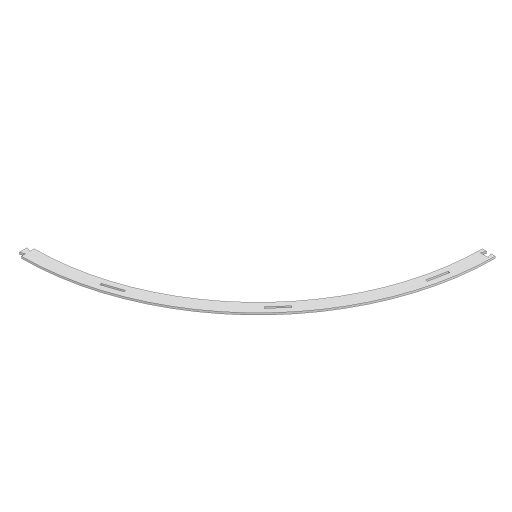
# Autodesk Inventor part: R70_CM_CIRCULO
Saved by Autodesk Inventor 2024.2 (Build 282272000, 272)
## iProperties
Created: 2024-10-01
Part Number: R70_CM_CIRCULO
Material: Generic
Document SubType Name: Modeling
Designer: jrcer
Density: 1 g/cm^3
Appearance: Default
Author: jrcer
Autodesk Inventor part; units mm, degrees
ref_plane "YZ Plane" through (0, 0, 0) normal (1, 0, 0) x (0, 1, 0)
ref_plane "XZ Plane" through (0, 0, 0) normal (0, 1, 0) x (-1, 0, 0)
ref_plane "XY Plane" through (0, 0, 0) normal (0, 0, 1) x (1, 0, 0)
sketch "Sketch1" plane through (0, 0, 0) normal (0, 1, 0) x (-1, 0, 0)
  circle A0 centre (0, 0) radius 350
  circle A1 centre (0, 0) radius 370
  line L0 (370, 0) -> (350, 0)
  line L1 (-370, 0) -> (-350, 0)
  line L2 (0, 0) -> (-350, 0) construction
  line L3 (0, 350) -> (0, 0) construction
  line L4 (0, 370) -> (0, 350)
  line L5 (-350, 0) -> (-370, 0)
  line L6 (-354, 7) -> (-366, 7)
  line L7 (-366, 7) -> (-363.4522, 0)
  line L8 (-354, 7) -> (-356.5478, 0)
  line L9 (-360, 0) -> (-360, 7) construction
  line L10 (-356.9749, 57.6407) -> (-350.9683, 87.0332)
  line L11 (-350.9683, 87.0332) -> (-347.8331, 86.3925)
  line L12 (-347.8331, 86.3925) -> (-353.8397, 57)
  line L13 (-353.8397, 57) -> (-356.9749, 57.6407)
  line L14 (-356.9749, 57.6407) -> (-347.8331, 86.3925) construction
  line L15 (-350.9683, 87.0332) -> (-353.8397, 57) construction
  circle A2 centre (0, 0) radius 360 construction
  line L16 (-7, -354) -> (0, -356.5478)
  line L17 (-7, -366) -> (0, -363.4522)
  line L18 (-7, -354) -> (-7, -366)
  line L19 (354, -7) -> (356.5478, 0)
  line L20 (366, -7) -> (363.4522, 0)
  line L21 (354, -7) -> (366, -7)
  line L22 (7, 354) -> (0, 356.5478)
  line L23 (7, 366) -> (0, 363.4522)
  line L24 (7, 354) -> (7, 366)
  line L25 (-337.9697, -128.5692) -> (-347.4641, -100.1112)
  line L26 (-334.9342, -127.5564) -> (-337.9697, -128.5692)
  line L27 (-344.4286, -99.0984) -> (-334.9342, -127.5564)
  line L28 (-347.4641, -100.1112) -> (-344.4286, -99.0984)
  line L29 (-228.4058, -280.329) -> (-250.8572, -260.4309)
  line L30 (-226.2833, -277.9342) -> (-228.4058, -280.329)
  line L31 (-248.7347, -258.0361) -> (-226.2833, -277.9342)
  line L32 (-250.8572, -260.4309) -> (-248.7347, -258.0361)
  line L33 (-57.6407, -356.9749) -> (-87.0332, -350.9683)
  line L34 (-57, -353.8397) -> (-57.6407, -356.9749)
  line L35 (-86.3925, -347.8331) -> (-57, -353.8397)
  line L36 (-87.0332, -350.9683) -> (-86.3925, -347.8331)
  line L37 (128.5692, -337.9697) -> (100.1112, -347.4641)
  line L38 (127.5564, -334.9342) -> (128.5692, -337.9697)
  line L39 (99.0984, -344.4286) -> (127.5564, -334.9342)
  line L40 (100.1112, -347.4641) -> (99.0984, -344.4286)
  line L41 (280.329, -228.4058) -> (260.4309, -250.8572)
  line L42 (277.9342, -226.2833) -> (280.329, -228.4058)
  line L43 (258.0361, -248.7347) -> (277.9342, -226.2833)
  line L44 (260.4309, -250.8572) -> (258.0361, -248.7347)
  line L45 (356.9749, -57.6407) -> (350.9683, -87.0332)
  line L46 (353.8397, -57) -> (356.9749, -57.6407)
  line L47 (347.8331, -86.3925) -> (353.8397, -57)
  line L48 (350.9683, -87.0332) -> (347.8331, -86.3925)
  line L49 (337.9697, 128.5692) -> (347.4641, 100.1112)
  line L50 (334.9342, 127.5564) -> (337.9697, 128.5692)
  line L51 (344.4286, 99.0984) -> (334.9342, 127.5564)
  line L52 (347.4641, 100.1112) -> (344.4286, 99.0984)
  line L53 (228.4058, 280.329) -> (250.8572, 260.4309)
  line L54 (226.2833, 277.9342) -> (228.4058, 280.329)
  line L55 (248.7347, 258.0361) -> (226.2833, 277.9342)
  line L56 (250.8572, 260.4309) -> (248.7347, 258.0361)
  line L57 (57.6407, 356.9749) -> (87.0332, 350.9683)
  line L58 (57, 353.8397) -> (57.6407, 356.9749)
  line L59 (86.3925, 347.8331) -> (57, 353.8397)
  line L60 (87.0332, 350.9683) -> (86.3925, 347.8331)
  line L61 (-128.5692, 337.9697) -> (-100.1112, 347.4641)
  line L62 (-127.5564, 334.9342) -> (-128.5692, 337.9697)
  line L63 (-99.0984, 344.4286) -> (-127.5564, 334.9342)
  line L64 (-100.1112, 347.4641) -> (-99.0984, 344.4286)
  line L65 (-280.329, 228.4058) -> (-260.4309, 250.8572)
  line L66 (-277.9342, 226.2833) -> (-280.329, 228.4058)
  line L67 (-258.0361, 248.7347) -> (-277.9342, 226.2833)
  line L68 (-260.4309, 250.8572) -> (-258.0361, 248.7347)
  point P0 (360, 0)
  point P1 (-360, 0)
  point P2 (-352.404, 72.0166)
  point P3 (-68.8261, 353.3595)
  point P4 (-355.4073, 57.3204)
  point P5 (-349.4007, 86.7129)
  point P6 (-7, -360)
  point P7 (360, -7)
  point P8 (7, 360)
  point P9 (-336.452, -128.0628)
  point P10 (-345.9464, -99.6048)
  point P11 (-227.3446, -279.1316)
  point P12 (-249.7959, -259.2335)
  point P13 (-57.3204, -355.4073)
  point P14 (-86.7129, -349.4007)
  point P15 (128.0628, -336.452)
  point P16 (99.6048, -345.9464)
  point P17 (279.1316, -227.3446)
  point P18 (259.2335, -249.7959)
  point P19 (355.4073, -57.3204)
  point P20 (349.4007, -86.7129)
  point P21 (336.452, 128.0628)
  point P22 (345.9464, 99.6048)
  point P23 (227.3446, 279.1316)
  point P24 (249.7959, 259.2335)
  point P25 (57.3204, 355.4073)
  point P26 (86.7129, 349.4007)
  point P27 (-128.0628, 336.452)
  point P28 (-99.6048, 345.9464)
  point P29 (-279.1316, 227.3446)
  point P30 (-259.2335, 249.7959)
  point P31 (0, 356.5478)
  point P32 (0, 363.4522)
  dimension "d0" = 700
  dimension "d1" = 740
  dimension "d4" = 90
  dimension "d5" = 7
  dimension "d6" = 70
  dimension "d8" = 12
  dimension "d13" = 3.2
  dimension "d14" = 30
  dimension "d15" = 50
  dimension "d20" = 720
  dimension "d23" = 360
  dimension "d27" = 360
  constraints: 138 end point, 11 point on circle, 8 midpoint, 3 centre point, 3 coincident, 3 parallel, 2 horizontal, 2 horizontal alignment, 2 perpendicular, 2 point on line, 2 vertical, 1 collinear, 1 equal length, 154 other
  measures "d0" diameter of A0
  measures "d1" diameter of A1
  measures "d4" angle of L2 L3
  measures "d5" distance between parallel lines of L6 L5
  measures "d6" angle of L7 L6
  measures "d8" distance of L6.start L6.end
  measures "d13" distance of L10.end L11.end
  measures "d14" distance of L11.end L12.end
  measures "d15" vertical distance of L12.end L6.start
  measures "d20" diameter of A2
extrude "Extrusion1" add sketch "Sketch1" along normal blind 3 contours A0 L1 L8 L6 L7 A1 L4 | L4 L23 L24 L22
body "Solid1"
